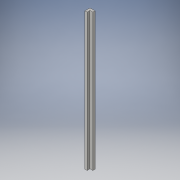
# Autodesk Inventor part: Molding 4 ft 5 3_4 in
Saved by Autodesk Inventor 2016 (Build 200138000, 138)
## iProperties
Created: 2015-05-31
Part Number: Molding 4 ft 5 3_4 in
Material: Generic
Document SubType Name: Modeling
Designer: steele
Density: 1 g/cm^3
Appearance: Default
Author: steele
Autodesk Inventor part; units mm, degrees
ref_plane "YZ Plane" through (0, 0, 0) normal (1, 0, 0) x (0, 1, 0)
ref_plane "XZ Plane" through (0, 0, 0) normal (0, 1, 0) x (-1, 0, 0)
ref_plane "XY Plane" through (0, 0, 0) normal (0, 0, 1) x (1, 0, 0)
sketch "Sketch1" plane through (0, 0, 0) normal (0, 1, 0) x (-1, 0, 0)
  line L0 (0, -50.8) -> (50.8, -50.8)
  line L1 (50.8, -50.8) -> (50.8, 0)
  line L2 (-50.8, 50.8) -> (50.8, -50.8) construction
  line L3 (-50.8, -50.8) -> (50.8, 50.8) construction
  line L4 (0, -28.575) -> (28.575, -28.575)
  line L5 (28.575, -28.575) -> (28.575, 0)
  line L6 (-28.575, 28.575) -> (28.575, -28.575) construction
  line L7 (-28.575, -28.575) -> (28.575, 28.575) construction
  line L8 (50.8, 0) -> (28.575, 0)
  line L9 (0, -28.575) -> (0, -50.8)
  point P0 (0, 0)
  dimension "d2" = 50.8
  constraints: 20 end point, 4 midpoint
  measures "d2" distance from line of L9 L0.end
extrude "Extrusion1" add sketch "Sketch1" along normal blind 1365.25
body "Solid1"
